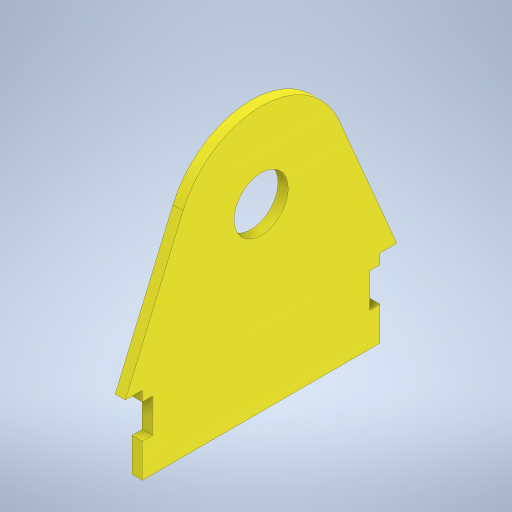
# Autodesk Inventor part: baseSoporte2
Saved by Autodesk Inventor 2024.3 (Build 283343000, 343)
## iProperties
Created: 2024-05-14
Part Number: baseSoporte2
Material: PMMA Plastic
Document SubType Name: Modeling
Designer: USUARIO
Density: 1.188 g/cm^3
Appearance: Canary
Mass: 15.1746 g
Surface Area: 94.6312 cm^2
Volume: 12.7732 cm^3
Author: USUARIO
Autodesk Inventor part; units mm, degrees
ref_plane "YZ Plane" through (0, 0, 0) normal (1, 0, 0) x (0, 1, 0)
ref_plane "XZ Plane" through (0, 0, 0) normal (0, 1, 0) x (-1, 0, 0)
ref_plane "XY Plane" through (0, 0, 0) normal (0, 0, 1) x (1, 0, 0)
sketch "Sketch1" plane through (0, 0, 0) normal (1, 0, 0) x (0, 1, 0)
  circle A0 centre (0, 0) radius 8
  arc A1 (-25, 0) -> (9.8205, -22.9904) centre (0, 0) ccw construction
  line L0 (0, 0) -> (-30, 0) construction
  line L1 (-30, 0) -> (-30, -35) construction
  line L2 (-30, -40) -> (9.8205, -22.9904)
  line L3 (-30, 0) -> (-30, 35) construction
  line L4 (-30, 40) -> (9.8205, 22.9904)
  line L5 (-30, 0) -> (-33, 0) construction
  line L6 (-33, 0) -> (-33, -35) construction
  line L7 (-33, -35) -> (-30, -35)
  line L8 (-33, 0) -> (-33, 32) construction
  line L9 (-33, 35) -> (-30, 35)
  line L10 (-33, 35) -> (-43, 35) construction
  line L11 (-43, 35) -> (-43, -32) construction
  line L12 (-43, -35) -> (-33, -35) construction
  line L13 (-33, -35) -> (-33, -32)
  line L14 (-33, 35) -> (-43, 35) construction
  line L15 (-43, 35) -> (-43, 32)
  line L16 (-43, 32) -> (-33, 32)
  line L17 (-33, 32) -> (-33, 35)
  line L18 (-43, -35) -> (-33, -35) construction
  line L19 (-33, -35) -> (-33, -32)
  line L20 (-33, -32) -> (-43, -32)
  line L21 (-43, -32) -> (-43, -35)
  line L22 (-43, 35) -> (-46, 35)
  line L23 (-46, 35) -> (-46, -35) construction
  line L24 (-46, -35) -> (-43, -35)
  line L25 (-43, -35) -> (-43, -32)
  arc A2 (9.8205, 22.9904) -> (-25, 0) centre (0, 0) ccw construction
  arc A3 (9.8205, -22.9904) -> (9.8205, 22.9904) centre (0, 0) ccw
  line L26 (-30, 35) -> (-30, 40)
  line L27 (-30, -35) -> (-30, -40)
  line L28 (-33, 32) -> (-33, 35)
  line L29 (-33, -32) -> (-33, 35) construction
  line L30 (-43, -32) -> (-43, -35)
  line L31 (-43, 32) -> (-43, 35)
  line L32 (-43, -32) -> (-43, 32) construction
  line L33 (-46, 35) -> (-53, 35)
  line L34 (-53, 35) -> (-53, -35)
  line L35 (-53, -35) -> (-46, -35)
  point P0 (-43, -25)
  dimension "d0" = 16
  dimension "d1" = 50
  dimension "d2" = 30
  dimension "d4" = 40
  dimension "d5" = 40
  dimension "d8" = 3
  dimension "d19" = 10
  dimension "d20" = 70
  dimension "d21" = 3
  dimension "d22" = 3
  dimension "d23" = 3
  dimension "d24" = 35
  dimension "d25" = 7
  dimension "d26" = 70
  dimension "d27" = 7
  constraints: 72 end point, 13 parallel, 11 perpendicular, 7 horizontal, 6 point on circle, 4 centre point, 4 point on line, 4 tangent, 2 coincident, 2 vertical
  measures "d0" diameter of A0
  measures "d1" diameter of A1
  measures "d2" distance of L0.start L0.end
  measures "d4" distance of L0.end L2.start
  measures "d5" distance of L0.end L4.start
  measures "d8" distance of L0.end L5.end
  measures "d19" distance of L6.end L12.start
  measures "d20" distance of L12.start L10.end
  measures "d21" distance of L15.end L14.end
  measures "d22" distance of L13.end L18.end
  measures "d23" distance of L12.start L23.end
  measures "d24" distance of L5.end L6.end
  measures "d25" distance of L22.end L33.end
  measures "d26" distance of L33.end L34.end
  measures "d27" distance of L34.end L23.end
extrude "Extrusion1" add sketch "Sketch1" along normal blind 3
body "Solid1"
